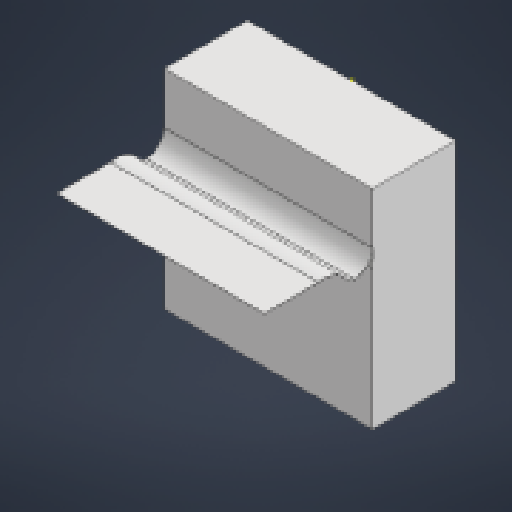
# Autodesk Inventor part: 便签
Saved by Autodesk Inventor 2025 (Build 290162000, 162)
## iProperties
Created: 2025-11-30
Part Number: 便签
Material: 常规
Document SubType Name: Modeling
Designer: XH
Density: 1 g/cm^3
Appearance: 默认
Author: XH
Autodesk Inventor part; units mm, degrees
ref_plane "YZ Plane" through (0, 0, 0) normal (1, 0, 0) x (0, 1, 0)
ref_plane "XZ Plane" through (0, 0, 0) normal (0, 1, 0) x (-1, 0, 0)
sketch "草图1" plane through (0, 0, 0) normal (0, 0, 1) x (1, 0, 0)
  line L0 (37.5, -37.5) -> (-37.5, -37.5)
  line L1 (-37.5, -37.5) -> (-37.5, 37.5)
  line L2 (-37.5, 37.5) -> (37.5, 37.5)
  line L3 (37.5, 37.5) -> (37.5, -37.5)
  line L4 (37.5, -37.5) -> (-37.5, 37.5) construction
  line L5 (-37.5, -37.5) -> (37.5, 37.5) construction
  point P0 (0, 0)
  dimension "d0" = 75
  dimension "d1" = 75
  constraints: 12 end point, 2 midpoint, 2 parallel, 1 horizontal, 1 perpendicular
  measures "d0" distance of L1.end L2.end
  measures "d1" distance of L2.end L0.start
extrude "拉伸1" add sketch "草图1" along normal blind 30
sketch "草图2" plane through (-37.5, 37.5, 0) normal (0, 1, 0) x (1, 0, 0)
  point P0 (37.5, 0)
ref_plane "工作平面1" through (-37.5, 12.5, 0) normal (0, 1, 0) x (1, 0, 0)
sketch "草图3" plane through (-37.5, 12.5, 0) normal (0, 1, 0) x (1, 0, 0)
  line L0 (75, -30) -> (0, -30) projected
  line L1 (75, -30) -> (0, -30)
  line L2 (0, -30) -> (0, -80)
  line L3 (0, -80) -> (75, -80)
  line L4 (75, -80) -> (75, -30)
  line L5 (0, 0) -> (0, -30) projected
  point P0 (37.5, 0)
  dimension "d5" = 50
  constraints: 8 end point, 2 parallel, 1 collinear, 1 horizontal, 1 perpendicular
  measures "d5" distance between parallel lines of L0 L3
extrude "拉伸2" add sketch "草图3" along normal blind 0.1
fillet "圆角1" radius 6.5 1 edges at (0, 12.6, 30)
sketch "草图4" plane through (-37.5, -37.5, 0) normal (-1, 0, 0) x (0, 0, 1)
  arc A0 (30, 56.6) -> (36.5, 50.1) centre (36.5, 56.6) ccw projected
  circle A1 centre (36.5, 56.6) radius 6.6
  line L0 (80, 50) -> (30, 50) projected
  line L1 (30, 50) -> (29.9, 56.6)
  point P0 (0, 37.5)
  point P1 (29.90303, 56.400046)
  point P2 (36.5, 50)
  constraints: 2 end point, 1 coincident, 1 horizontal, 3 other
extrude "拉伸3" cut sketch "草图4" against normal blind 112.5 contours A1 L0 L1
sketch "草图5" plane through (-37.5, 12.6, 0) normal (0, 1, 0) x (1, 0, 0)
  line L0 (0, -36.5) -> (75, -36.5) projected
  line L1 (0, -36.5) -> (0, -80) projected
  line L2 (0, -80) -> (75, -80) projected
  line L3 (75, -80) -> (75, -36.5) projected
  point P0 (37.5, 0)
extrude "拉伸4" cut sketch "草图5" against normal blind 10
sketch "草图6" plane through (37.5, -37.5, 0) normal (1, 0, 0) x (0, 0, -1)
  circle A0 centre (-36.290069, 53.867726) radius 3.77357
  circle A1 centre (-36.290069, 53.867726) radius 3.873419
  circle A2 centre (-47.408546, 45.749477) radius 9.893293
  circle A3 centre (-47.408546, 45.749477) radius 9.993293
  line L0 (-49.395081, 55.441273) -> (-68.85686, 55.441273)
  line L1 (-68.85686, 55.441273) -> (-68.85686, 55.541273)
  line L2 (-68.85686, 55.541273) -> (-49.395081, 55.541273)
  line L3 (-49.395081, 55.541273) -> (-49.395081, 55.441273)
  line L4 (-36.5, 50) -> (-36.5, 50.1)
  line L5 (-39.337702, 51.642471) -> (-41.290421, 53.524165)
  point P0 (0, 37.5)
  point P1 (-49.405198, 55.541273)
  point P2 (-39.653725, 51.947)
  dimension "d13" = 0.1
  constraints: 12 end point, 4 point on circle, 2 centre point, 2 coincident, 2 parallel, 1 horizontal, 1 perpendicular, 1 vertical, 7 other
sketch "草图6 outline for 拉伸5" plane through (37.5, -37.5, 0) normal (1, 0, 0) x (0, 0, -1)
  line L0 (-36.5, 50) -> (-36.5, 50.1)
  arc A0 (-39.653725, 51.947) -> (-36.5, 50) centre (-36.290069, 53.867726) ccw
  line L1 (-41.290421, 53.524165) -> (-39.653725, 51.947)
  arc A1 (-49.395081, 55.441273) -> (-41.290421, 53.524165) centre (-47.408546, 45.749477) cw
  line L2 (-68.85686, 55.441273) -> (-49.395081, 55.441273)
  line L3 (-68.85686, 55.541273) -> (-68.85686, 55.441273)
  line L4 (-49.405198, 55.541273) -> (-68.85686, 55.541273)
  arc A2 (-39.337702, 51.642471) -> (-49.405198, 55.541273) centre (-47.408546, 45.749477) ccw
  arc A3 (-36.5, 50.1) -> (-39.337702, 51.642471) centre (-36.290069, 53.867726) cw
extrude "拉伸5" add sketch "草图6 outline for 拉伸5" against normal up to surface (75 mm away)
